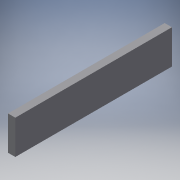
# Autodesk Inventor part: Short-Brace
Saved by Autodesk Inventor 2017 (Build 210142000, 142)
## iProperties
Created: 2017-08-30
Part Number: Short-Brace
Material: Generic
Document SubType Name: Modeling
Designer: Trent
Density: 1 g/cm^3
Appearance: Yellow Pine - Solid Stained Light Low Gloss
Author: Trent
Autodesk Inventor part; units mm, degrees
ref_plane "YZ Plane" through (0, 0, 0) normal (1, 0, 0) x (0, 1, 0)
ref_plane "XZ Plane" through (0, 0, 0) normal (0, 1, 0) x (-1, 0, 0)
ref_plane "XY Plane" through (0, 0, 0) normal (0, 0, 1) x (1, 0, 0)
sketch "Sketch1" plane through (0, 0, 0) normal (1, 0, 0) x (0, 1, 0)
  line L0 (-44.45, 204.7875) -> (44.45, 204.7875)
  line L1 (44.45, 204.7875) -> (44.45, -204.7875)
  line L2 (44.45, -204.7875) -> (-44.45, -204.7875)
  line L3 (-44.45, -204.7875) -> (-44.45, 204.7875)
  line L4 (-44.45, 204.7875) -> (44.45, -204.7875) construction
  line L5 (44.45, 204.7875) -> (-44.45, -204.7875) construction
  point P0 (0, 0)
  dimension "d0" = 88.9
  dimension "d1" = 409.575
  constraints: 12 end point, 2 midpoint, 2 parallel, 1 horizontal, 1 perpendicular
  measures "d0" distance of L1.end L2.end
  measures "d1" distance of L0.end L1.end
extrude "Extrusion1" add sketch "Sketch1" along normal blind 19.05
body "Solid1"
